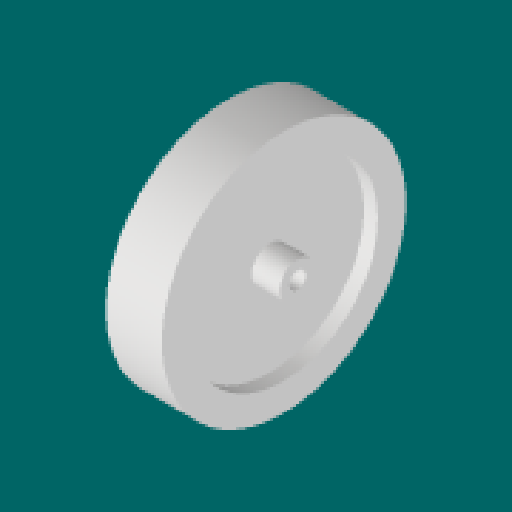
# Autodesk Inventor part: PK
Saved by Autodesk Inventor 2023 (Build 270158000, 158)
## iProperties
Created: 2023-01-04
Part Number: PK
Material: Generic
Document SubType Name: Modeling
Designer: HeavyDrewno
Density: 1 g/cm^3
Appearance: Default
Author: HeavyDrewno
Autodesk Inventor part; units mm, degrees
ref_plane "YZ Plane" through (0, 0, 0) normal (1, 0, 0) x (0, 1, 0)
ref_plane "XZ Plane" through (0, 0, 0) normal (0, 1, 0) x (-1, 0, 0)
ref_plane "XY Plane" through (0, 0, 0) normal (0, 0, 1) x (1, 0, 0)
sketch "Sketch1" plane through (0, 0, 0) normal (0, 1, 0) x (-1, 0, 0)
  line L0 (0, 0) -> (30, 0) construction
  line L1 (30, 0) -> (30, -6) construction
  line L2 (30, -6) -> (30, -13)
  line L3 (0, -87.5) -> (20, -87.5)
  line L4 (20, -87.5) -> (20, -67.5)
  line L5 (30, -6) -> (0, -6)
  line L6 (0, 0) -> (0, -87.5) construction
  line L7 (0, 0) -> (-30, 0) construction
  line L8 (-30, 0) -> (-30, -6) construction
  line L9 (-30, -6) -> (-30, -13)
  line L10 (0, -87.5) -> (-20, -87.5)
  line L11 (-20, -87.5) -> (-20, -67.5)
  line L12 (-30, -6) -> (0, -6)
  line L13 (20, -67.5) -> (10, -67.5)
  line L14 (10, -67.5) -> (10, -13)
  line L15 (10, -13) -> (30, -13)
  line L16 (-10, -67.5) -> (-10, -13)
  line L17 (-10, -13) -> (-30, -13)
  line L18 (-20, -67.5) -> (-10, -67.5)
  dimension "d0" = 30
  dimension "d1" = 6
  dimension "d3" = 7
  dimension "d4" = 20
  dimension "d5" = 87.5
  dimension "d6" = 20
  dimension "d8" = 10
  constraints: 38 end point, 7 symmetric about line, 5 horizontal, 4 vertical, 2 perpendicular
  measures "d0" distance of L0.start L0.end
  measures "d1" distance of L0.end L1.end
  measures "d3" distance of L1.end L2.end
  measures "d4" distance of L3.start L3.end
  measures "d5" distance between parallel lines of L3 L0
  measures "d6" distance of L3.end L4.end
  measures "d8" distance of L4.end L13.end
revolve "Revolution1" add sketch "Sketch1" angle 360 about axis through (0, 0, 0) along (1, 0, 0)
body "Solid1"
